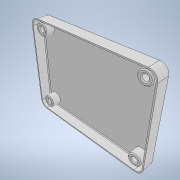
# Autodesk Inventor part: Корпус платы
Saved by Autodesk Inventor 2021.1 (Build 251245010, 245A)
## iProperties
Created: 2026-06-02
Part Number: Корпус платы
Material: Типовые
Document SubType Name: Modeling
Designer: Андрей Тарасов
Density: 1 g/cm^3
Appearance: По умолчанию
Author: Андрей Тарасов
Autodesk Inventor part; units mm, degrees
ref_plane "YZ Plane" through (0, 0, 0) normal (1, 0, 0) x (0, 1, 0)
ref_plane "XZ Plane" through (0, 0, 0) normal (0, 1, 0) x (-1, 0, 0)
ref_plane "XY Plane" through (0, 0, 0) normal (0, 0, 1) x (1, 0, 0)
sketch "Эскиз1" plane through (0, 0, 0) normal (0, 0, 1) x (1, 0, 0)
  line L0 (5, 0) -> (75, 0)
  line L1 (80, 5) -> (80, 55)
  line L2 (75, 60) -> (5, 60)
  line L3 (0, 55) -> (0, 5)
  arc A0 (5, 60) -> (0, 55) centre (5, 55) ccw
  arc A1 (80, 55) -> (75, 60) centre (75, 55) ccw
  arc A2 (0, 5) -> (5, 0) centre (5, 5) ccw
  arc A3 (75, 0) -> (80, 5) centre (75, 5) ccw
  point P0 (0, 0)
  point P1 (80, 60)
  point P2 (80, 0)
  point P3 (0, 60)
  dimension "d0" = 60
  dimension "d1" = 80
  dimension "d14" = 5
  constraints: 8 end point, 8 point on circle, 8 point on line, 8 tangent, 4 centre point, 3 equal radius, 2 parallel, 1 horizontal, 1 perpendicular
  measures "d0" distance of point (0, 60) point (0, 0)
  measures "d1" distance of point (0, 0) point (80, 0)
  measures "d14" radius of A0
extrude "Выдавливание1" add sketch "Эскиз1" along normal blind 1
sketch "Эскиз2" plane through (0, 0, 1) normal (0, 0, 1) x (1, 0, 0)
  line L0 (80, 5) -> (80, 55) projected
  line L1 (75, 60) -> (5, 60) projected
  line L2 (0, 55) -> (0, 5) projected
  line L3 (5, 0) -> (75, 0) projected
  line L4 (0, 60) -> (0, 0) projected
  line L5 (0, 54) -> (80, 54) construction
  line L6 (80, 0) -> (80, 60) projected
  line L7 (0, 6) -> (80, 6) construction
  line L8 (6.5, 60) -> (6.5, 0) construction
  line L9 (0, 0) -> (80, 0) projected
  line L10 (80, 60) -> (0, 60) projected
  line L11 (73.5, 60) -> (73.5, 0) construction
  line L12 (0, 0) -> (80, 0) projected
  circle A0 centre (6.5, 54) radius 4
  circle A1 centre (73.5, 54) radius 4
  circle A2 centre (6.5, 6) radius 4
  circle A3 centre (73.5, 6) radius 4
  circle A4 centre (6.5, 54) radius 1.75
  circle A5 centre (73.5, 54) radius 1.75
  circle A6 centre (6.5, 6) radius 1.75
  circle A7 centre (73.5, 6) radius 1.75
  arc A8 (0, 5) -> (5, 0) centre (5, 5) ccw projected
  arc A9 (75, 0) -> (80, 5) centre (75, 5) ccw projected
  arc A10 (80, 55) -> (75, 60) centre (75, 55) ccw projected
  arc A11 (5, 60) -> (0, 55) centre (5, 55) ccw projected
  dimension "d4" = 48
  dimension "d5" = 67
  dimension "d6" = 6
  dimension "d7" = 6.5
  dimension "d8" = 8
  dimension "d10" = 3.5
  constraints: 16 point on line, 8 centre point, 8 end point, 6 equal radius, 4 coincident, 4 perpendicular
  measures "d4" distance between parallel lines of L7 L5
  measures "d5" distance between parallel lines of L11 L8
  measures "d6" distance between parallel lines of L12 L7
  measures "d7" distance between parallel lines of L2 L8
  measures "d8" diameter of A0
  measures "d10" diameter of A4
extrude "Выдавливание2" add sketch "Эскиз2" along normal blind 6 contours A0 | A1 | A2 | A3
sketch "Эскиз3" plane through (0, 0, 1) normal (0, 0, 1) x (1, 0, 0)
  circle A0 centre (6.5, 6) radius 4 projected
  circle A1 centre (73.5, 54) radius 4 projected
  circle A2 centre (73.5, 6) radius 4 projected
  circle A3 centre (6.5, 54) radius 4 projected
  line L0 (0, 55) -> (0, 5) projected
  arc A4 (0, 5) -> (5, 0) centre (5, 5) ccw projected
  line L1 (5, 0) -> (75, 0) projected
  arc A5 (75, 0) -> (80, 5) centre (75, 5) ccw projected
  line L2 (80, 5) -> (80, 55) projected
  arc A6 (80, 55) -> (75, 60) centre (75, 55) ccw projected
  line L3 (75, 60) -> (5, 60) projected
  arc A7 (5, 60) -> (0, 55) centre (5, 55) ccw projected
  line L4 (5, 59.2) -> (75, 59.2)
  arc A8 (79.2, 55) -> (75, 59.2) centre (75, 55) ccw
  line L5 (79.2, 55) -> (79.2, 5)
  arc A9 (75, 0.8) -> (79.2, 5) centre (75, 5) ccw
  line L6 (75, 0.8) -> (5, 0.8)
  arc A10 (0.8, 5) -> (5, 0.8) centre (5, 5) ccw
  line L7 (0.8, 5) -> (0.8, 55)
  arc A11 (5, 59.2) -> (0.8, 55) centre (5, 55) ccw
  line L8 (6.5, 50) -> (0.8, 50)
  circle A12 centre (6.5, 54) radius 4 projected
  line L9 (10.5, 54) -> (10.5, 59.2)
  line L10 (0.8, 10) -> (6.5, 10)
  circle A13 centre (6.5, 6) radius 4 projected
  line L11 (10.5, 0.8) -> (10.5, 6)
  line L12 (69.5, 0.8) -> (69.5, 6)
  circle A14 centre (73.5, 6) radius 4 projected
  circle A15 centre (73.5, 6) radius 4 projected
  line L13 (73.5, 10) -> (79.2, 10)
  circle A16 centre (73.5, 54) radius 4 projected
  line L14 (73.5, 50) -> (79.2, 50)
  line L15 (69.5, 59.2) -> (69.5, 54)
  point P0 (0, 0)
  dimension "d15" = 0.8
  constraints: 24 end point, 11 point on circle, 11 point on line, 7 perpendicular, 4 centre point, 4 tangent, 3 horizontal alignment, 2 vertical alignment, 1 horizontal, 1 vertical, 12 other
  measures "d15" distance between parallel lines of L3 L4
extrude "Выдавливание3" add sketch "Эскиз3" along normal blind 7
chamfer "Фаска1" distance 0.6 angle 45 24 edges at (40, 0, 0) (78.5355, 1.4645, 0) (80, 30, 0) (78.5355, 58.5355, 0) (40, 60, 0) (1.4645, 58.5355, 0) (0, 30, 0) (1.4645, 1.4645, 0) (40, 59.2, 1) (2.0302, 57.9698, 1) (0.8, 30, 1) (2.0302, 2.0302, 1) (40, 0.8, 1) (77.9698, 2.0302, 1) (79.2, 30, 1) (77.9698, 57.9698, 1) (4.75, 6, 7) (2.5, 6, 7) (4.75, 54, 7) (2.5, 54, 7) (71.75, 54, 7) (69.5, 54, 7) (71.75, 6, 7) (69.5, 6, 7)
